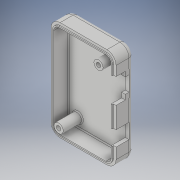
# Autodesk Inventor part: Top
Saved by Autodesk Inventor 2018.3 (Build 223284000, 284)
## iProperties
Created: 2018-10-08
Part Number: Top
Material: Generic
Document SubType Name: Modeling
Designer: birtj
Density: 1 g/cm^3
Appearance: Default
Author: birtj
Autodesk Inventor part; units mm, degrees
ref_plane "YZ Plane" through (0, 0, 0) normal (1, 0, 0) x (0, 1, 0)
ref_plane "XZ Plane" through (0, 0, 0) normal (0, 1, 0) x (-1, 0, 0)
ref_plane "XY Plane" through (0, 0, 0) normal (0, 0, 1) x (1, 0, 0)
sketch "OBJECT" plane through (0, 0, 0) normal (0, 0, 1) x (1, 0, 0)
  line L0 (177.8812, 243.8295) -> (177.8812, 295.7471)
  arc A0 (183.6724, 301.5383) -> (177.8812, 295.7471) centre (183.6724, 295.7471) ccw
  line L1 (183.6724, 301.5383) -> (213.492, 301.5383)
  arc A1 (219.2832, 295.7471) -> (213.492, 301.5383) centre (213.492, 295.7471) ccw
  line L2 (219.2832, 295.7471) -> (219.2832, 243.8295)
  arc A2 (213.492, 238.0383) -> (219.2832, 243.8295) centre (213.492, 243.8295) ccw
  line L3 (213.492, 238.0383) -> (183.6724, 238.0383)
  arc A3 (177.8812, 243.8295) -> (183.6724, 238.0383) centre (183.6724, 243.8295) ccw
  dimension "d2" = 63.5
  dimension "d3" = 41.402
  dimension "d26" = 5.7912
  constraints: 8 end point, 8 point on circle, 4 centre point
  measures "d2" distance between parallel lines of L3 L1
  measures "d3" distance between parallel lines of L2 L0
  measures "d26" radius of A0
extrude "Extrusion1" add sketch "OBJECT" along normal blind 11.4046
shell "Shell1" thickness 2.3622 removed faces 1 at (191.6819, 261.1354, 11.4046)
sketch "Sketch4" plane through (183.6724, 240.4005, 2.3622) normal (0, 0, 1) x (1, 0, 0)
  line L0 (29.8196, 61.1378) -> (0, 61.1378) construction
  line L1 (14.9098, 61.1378) -> (14.9098, -2.3622) construction
  line L2 (0, -2.3622) -> (29.8196, -2.3622) construction
  line L3 (-5.7912, 55.3466) -> (-5.7912, 3.429) construction
  line L4 (-5.7912, 29.3878) -> (35.6108, 29.3878) construction
  line L5 (35.6108, 3.429) -> (35.6108, 55.3466) construction
  circle A0 centre (2.2098, 5.6388) radius 2.921
  circle A1 centre (27.6098, 53.1622) radius 2.921
  dimension "d11" = 5.842
  dimension "d12" = 5.842
  dimension "d23" = 12.7
  dimension "d25" = 12.7
  dimension "d37" = 23.7744
  dimension "d39" = 23.749
  constraints: 4 end point, 4 midpoint, 2 centre point, 2 coincident
  measures "d11" diameter of A0
  measures "d12" diameter of A1
  measures "d23" distance from line of L1 A0.centre
  measures "d25" distance from line of L1 A1.centre
  measures "d37" distance from line of L4 point (27.61, 53.162)
  measures "d39" distance from line of L4 point (2.21, 5.639)
extrude "Extrusion2" add sketch "Sketch4" along normal up to surface (9.0424 mm away)
sketch "Sketch5" plane through (211.2822, 198.5413, 11.4046) normal (0, 0, 1) x (1, 0, 0)
  circle A0 centre (0, 95.0214) radius 2.921 projected
  point P0 (-25.4, 47.498)
hole "Hole1" at (211.2822, 293.5627, 11.4046) at (185.8822, 246.0393, 11.4046) direction (0, 0, -1) diameter 2.8448 end through all
fillet "Fillet1" radius 3.175 8 edges at (217.587, 299.8421, 0) (198.5822, 301.5383, 0) (179.5774, 299.8421, 0) (177.8812, 269.7883, 0) (179.5774, 239.7345, 0) (198.5822, 238.0383, 0) (217.587, 239.7345, 0) (219.2832, 269.7883, 0)
sketch "Sketch6" plane through (219.2832, 243.8295, 11.4046) normal (1, 0, 0) x (0, 0, -1)
  line L0 (0, 0) -> (0, 51.9176) projected
  line L1 (0, 6.9088) -> (8.255, 6.9088)
  line L2 (8.255, 6.9088) -> (8.255, 16.4338)
  line L3 (8.255, 16.4338) -> (0, 16.4338)
  line L4 (0, 16.4338) -> (0, 6.9088)
  line L5 (8.2296, -5.7912) -> (0, -5.7912) projected
  line L6 (0, 51.9176) -> (0, 0) projected
  line L7 (0, 45.7708) -> (8.255, 45.7708)
  line L8 (8.255, 45.7708) -> (8.255, 29.8958)
  line L9 (8.255, 29.8958) -> (0, 29.8958)
  line L10 (0, 29.8958) -> (0, 45.7708)
  line L11 (8.2296, 57.7088) -> (0, 57.7088) projected
  point P0 (11.4046, -243.8295)
  dimension "d28" = 12.7
  dimension "d29" = 9.525
  dimension "d30" = 8.255
  dimension "d33" = 8.255
  dimension "d34" = 15.875
  dimension "d35" = 11.938
  constraints: 16 end point, 4 parallel, 2 horizontal, 2 perpendicular, 2 point on line
  measures "d28" distance between parallel lines of L1 L5
  measures "d29" distance between parallel lines of L1 L3
  measures "d30" distance of L2.end L3.end
  measures "d33" distance of L8.end L9.end
  measures "d34" distance of L7.end L8.end
  measures "d35" distance between parallel lines of L11 L7
extrude "Extrusion3" cut sketch "Sketch6" against normal blind 2.54
lip "Lip2" kind lip height 0.762 width 0.762 edges at (216.921, 266.9943, 11.4046) guide face at (217.7084, 269.238, 11.4046)
lip "Lip3" kind lip height 0.762 width 0.762 edges at (215.9167, 241.4048, 11.4046) (198.5822, 240.4005, 11.4046) (181.2478, 241.4048, 11.4046) (180.2434, 269.7883, 11.4046) (181.2478, 298.1718, 11.4046) (198.5822, 299.1761, 11.4046) (215.9167, 298.1718, 11.4046) (216.921, 292.6737, 11.4046) (216.921, 247.2839, 11.4046) guide face at (178.6686, 261.1354, 11.4046)
fillet "Fillet2" radius 0.635 10 edges at (182.9612, 246.0393, 2.3622) (208.3612, 293.5627, 2.3622) (181.2478, 298.1718, 2.3622) (180.2434, 269.7883, 2.3622) (181.2478, 241.4048, 2.3622) (198.5822, 240.4005, 2.3622) (215.9167, 241.4048, 2.3622) (216.921, 269.7883, 2.3622) (215.9167, 298.1718, 2.3622) (198.5822, 299.1761, 2.3622)
sketch "Sketch9" plane through (185.8822, 246.0393, 11.4046) normal (0, 0, 1) x (1, 0, 0)
  circle A0 centre (0, 0) radius 1.4224 projected
  circle A1 centre (0, 0) radius 2.921 projected
  circle A2 centre (25.4, 47.5234) radius 1.4224 projected
  circle A3 centre (25.4, 47.5234) radius 2.921 projected
extrude "Extrusion5" add sketch "Sketch9" along normal blind 3.1877
sketch "Sketch10" plane through (0, 0, 0) normal (0, 0, -1) x (-1, 0, 0)
  line L0 (-183.6724, 301.5383) -> (-213.492, 301.5383) projected
  line L1 (-219.2831, 260.2633) -> (-219.2831, 250.7383) projected
  line L2 (-213.492, 238.0383) -> (-183.6724, 238.0383) projected
  line L3 (-177.8812, 243.8295) -> (-177.8812, 295.7471) projected
  point P0 (0, 0)
  point P1 (-190.2002, 292.0133)
  dimension "d76" = 53.975
  dimension "d77" = 12.319
  measures "d76" distance from line of L2 point (-190.2, 292.013)
  measures "d77" distance from line of L3 point (-190.2, 292.013)
hole "Hole2" at (190.2002, 292.0133, 0) direction (0, 0, 1) diameter 5.05 end through all
sketch "Sketch11" plane through (219.2832, 295.7471, 11.4046) normal (1, 0, 0) x (0, 0, -1)
  line L0 (8.255, -6.1468) -> (8.255, -22.0218) projected
  line L1 (8.255, -6.1468) -> (5.8738, -6.1468)
  line L2 (5.8738, -6.1468) -> (5.8738, -9.3218)
  line L3 (5.8738, -9.3218) -> (8.255, -9.3218)
  line L4 (8.255, -9.3218) -> (8.255, -6.1468)
  line L5 (0, -22.0218) -> (8.255, -22.0218) projected
  line L6 (8.255, -22.0218) -> (5.8737, -22.0218)
  line L7 (5.8737, -22.0218) -> (5.8737, -18.8468)
  line L8 (5.8737, -18.8468) -> (8.255, -18.8468)
  line L9 (8.255, -18.8468) -> (8.255, -22.0218)
  point P0 (11.4046, -295.7471)
  dimension "d78" = 2.3813
  dimension "d79" = 3.175
  dimension "d80" = 2.3813
  dimension "d81" = 3.175
  constraints: 16 end point, 4 parallel, 2 horizontal, 2 perpendicular
  measures "d78" distance of L3.end L2.end
  measures "d79" distance of L2.end L1.end
  measures "d80" distance of L7.end L8.end
  measures "d81" distance of L6.end L7.end
extrude "Extrusion6" add sketch "Sketch11" against normal up to surface (2.3622 mm away)
body "Solid1"
